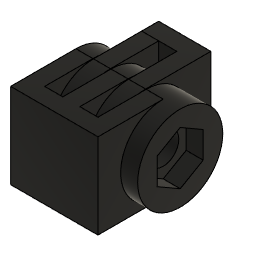
GoPro Profile (Autodesk Fusion 360 design; units mm, degrees)
Autodesk Fusion 360 part; units mm, degrees
ref_plane "WorkPlane1" through (-1.6, 0, 0) normal (1, 0, 0) x (0, 1, 0) in component "Gopro Profile Male"
sketch "Sketch25" plane through (-1.6, 0, 0) normal (1, 0, 0) x (0, 1, 0) in component "Gopro Profile Male"
  circle A0 centre (-8.5, 7.5) radius 7.5
  line L0 (0, 0) -> (-8.5, 0)
  line L1 (-0.0009, 15) -> (-8.5, 15)
  line L2 (-0.0009, 15) -> (0, 15)
  line L3 (0, 15) -> (0, 0)
  dimension "d499" = 15
  dimension "d631" = 8.5
  constraint coincident L0.start L3.end
  constraint coincident A0 L0.end
  constraint tangent A0 L0
  constraint horizontal L0
  constraint coincident A0 L1.end
  constraint tangent A0 L1
  constraint horizontal L1
  constraint vertical L3
  measures "d499" diameter of A0
  measures "d631" distance of A0.centre L3
extrude "Extrude16" add sketch "Sketch25" against normal blind 3 makes body 1 in component "Gopro Profile Male"
mirror "Mirror1" about plane through (0, 0, 0) normal (1, 0, 0) of "Extrude16" makes body 2 in component "Gopro Profile Male"
sketch "Sketch26" plane through (0, 0, 0) normal (0, 0, 1) x (1, 0, 0) in component "Gopro Profile Male"
  line L0 (-4.6, -0.0009) -> (4.6, -0.0009)
  line L1 (4.6, -0.0009) -> (4.6, 2.9991)
  line L2 (4.6, 2.9991) -> (-4.6, 2.9991)
  line L3 (-4.6, 2.9991) -> (-4.6, -0.0009)
  line L4 (4.6, -8.5) -> (4.6, -0.0009)
  point P0 (-4.6, -0.0009)
  dimension "d632" = 3
  constraint horizontal L0
  constraint vertical L1
  constraint horizontal L2
  constraint vertical L3
  constraint coincident P0 L0.start
  constraint collinear L1 L4
  measures "d632" distance of P0 L2.end
extrude "Extrude17" add sketch "Sketch26" along normal blind 15 bodies 1 2 in component "Gopro Profile Male"
hole "Hole4" at (-4.6, -8.5, 7.5) direction (1, 0, 0) diameter 5.5 depth 10 tip angle 118 bodies 1 in component "Gopro Profile Male"
sketch "Sketch1" plane through (0, 0, 0) normal (0, 0, 1) x (1, 0, 0) in component "Gopro Profile Female"
  line L0 (-1.6, -0.0009) -> (-1.6, -8.5)
  line L1 (-1.5, -1) -> (-1.5, -17)
  line L2 (-1.5, -17) -> (-4.7, -17)
  line L3 (-4.7, -17) -> (-4.7, -1)
  line L4 (-4.7, -1) -> (-7.7, -1)
  line L5 (-7.7, -1) -> (-7.7, -20)
  line L6 (-7.7, -20) -> (7.7, -20)
  line L7 (7.7, -20) -> (7.7, -1)
  line L8 (7.7, -1) -> (4.7, -1)
  line L9 (4.7, -1) -> (4.7, -17)
  line L10 (4.7, -17) -> (1.5, -17)
  line L11 (1.5, -17) -> (1.5, -1)
  line L12 (1.5, -1) -> (-1.5, -1)
  line L13 (7.7, -1) -> (10.7, -1)
  line L14 (10.7, -1) -> (10.7, -16)
  line L15 (10.7, -16) -> (4.7, -16)
  dimension "d509" = 3
  dimension "d510" = 1.5
  dimension "d511" = 3.2
  dimension "d512" = 17
  dimension "d513" = 16
  dimension "d514" = 3
  dimension "d525" = 15
  dimension "d526" = 3
  dimension "d615" = 3
  constraint parallel L0 L1
  constraint perpendicular L1 L2
  constraint perpendicular L2 L3
  constraint perpendicular L3 L4
  constraint perpendicular L4 L5
  constraint perpendicular L5 L6
  constraint perpendicular L6 L7
  constraint perpendicular L7 L8
  constraint perpendicular L6 L9
  constraint perpendicular L9 L10
  constraint collinear L4 L12
  constraint collinear L8 L12
  constraint collinear L2 L10
  constraint equal L2 L10
  constraint perpendicular L7 L13
  constraint perpendicular L13 L14
  constraint coincident L9 L15.end
  constraint perpendicular L9 L15
  constraint equal L4 L8
  constraint vertical L11
  measures "d509" distance of L1.start L11.end
  measures "d510" distance of origin L1
  measures "d511" distance of L1 L3
  measures "d512" distance of origin L2
  measures "d513" distance of L2 L12
  measures "d514" distance of L6 L10
  measures "d525" distance of L13.end L14.end
  measures "d526" distance of L7.end L13.end
  measures "d615" distance of L3.end L4.end
extrude "Extrude1" add sketch "Sketch1" along normal blind 15 separate body makes body 3 in component "Gopro Profile Female"
fillet "Fillet1" radius 7.5 8 edges at (-6.2, -1, 0) (7.7, -1, 0) (0, -1, 0) (-6.2, -1, 15) (0, -1, 15) (7.7, -1, 15) (9.2, -16, 15) (9.2, -16, 0) on bodies 3 in component "Gopro Profile Female"
hole "Hole1" at (-7.7, -8.5, 7.5) direction (1, 0, 0) diameter 5.5 depth 20 tip angle 118 bodies 3 in component "Gopro Profile Female"
sketch "Sketch4" plane through (10.7, 0, 0) normal (1, 0, 0) x (0, 1, 0) in component "Gopro Profile Female"
  circle A0 centre (-8.5, 7.5) radius 7.5
  line L0 (-4.45, 9.8383) -> (-8.5, 12.1765)
  line L1 (-8.5, 12.1765) -> (-12.55, 9.8383)
  line L2 (-12.55, 9.8383) -> (-12.55, 5.1617)
  line L3 (-12.55, 5.1617) -> (-8.5, 2.8235)
  line L4 (-8.5, 2.8235) -> (-4.45, 5.1617)
  line L5 (-4.45, 5.1617) -> (-4.45, 9.8383)
  circle A1 centre (-8.5, 7.5) radius 2.75
  point P0 (-8.5, 7.5)
  dimension "d527" = 8.1
  constraint coincident P0 A0.centre
  constraint vertical L2
  measures "d527" distance of L2 L5
extrude "Extrude3" cut sketch "Sketch4" against normal blind 3 contours L0 L1 L2 L3 L4 L5 | A1 bodies 3 in component "Gopro Profile Female"
sketch "Sketch6" plane through (0, 0, 15) normal (0, 0, 1) x (-1, 0, 0) in component "Gopro Profile Female"
  line L0 (-7.7, 8.5) -> (-4.7, 8.5)
  line L1 (-4.7, 8.5) -> (-4.7, 17)
  line L2 (-4.7, 17) -> (-1.5, 17)
  line L3 (-1.5, 17) -> (-1.5, 8.5)
  line L4 (-1.5, 8.5) -> (1.5, 8.5)
  line L5 (1.5, 8.5) -> (1.5, 17)
  line L6 (1.5, 17) -> (4.7, 17)
  line L7 (4.7, 17) -> (4.7, 8.5)
  line L8 (4.7, 8.5) -> (7.7, 8.5)
  line L9 (0, 20.4687) -> (5.6563, 23.7344)
  line L10 (5.6562, 23.7344) -> (5.6563, 30.2656)
  line L11 (5.6563, 30.2656) -> (0, 33.5313)
  line L12 (0, 33.5313) -> (-5.6562, 30.2656)
  line L13 (-5.6562, 30.2656) -> (-5.6563, 23.7344)
  line L14 (-5.6563, 23.7344) -> (0, 20.4687)
  line L15 (-7.7, 20) -> (-7.7, 8.5)
  line L16 (7.7, 8.5) -> (7.7, 20)
  line L17 (7.7, 20) -> (-7.7, 20)
  point P0 (0, 27)
  point P1 (0, 27)
  dimension "d534" = 11.3125
  constraint coincident P1 P0
  constraint vertical L13
  constraint vertical origin P1
  measures "d534" distance of L10 L13
hole "Hole2" at (0, -27, 15) direction (0, 0, -1) diameter 7.142 depth 20 tip angle 118 bodies 3 in component "Gopro Profile Female"
component "Gopro Profile Male" placed x (1, 0, 0) y (0, 1, 0) z (0, 0, 1) at (0, 0, 0)
component "Gopro Profile Female" placed x (1, 0, 0) y (0, 1, 0) z (0, 0, 1) at (0, 0, 0)
equation "d534 = 0.4375 in + 0.2 mm"
